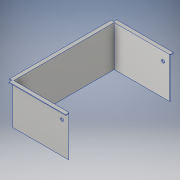
# Autodesk Inventor part: Intake Drop
Saved by Autodesk Inventor 2017 (Build 210142000, 142)
## iProperties
Created: 2020-02-19
Part Number: Intake Drop
Material: Aluminum 6061
Document SubType Name: Modeling
Designer: S346553810
Density: 2.7 g/cm^3
Appearance: Aluminum - Flat
Author: S346553810
Autodesk Inventor part; units mm, degrees
ref_plane "YZ Plane" through (0, 0, 0) normal (1, 0, 0) x (0, 1, 0)
ref_plane "XZ Plane" through (0, 0, 0) normal (0, 1, 0) x (-1, 0, 0)
ref_plane "XY Plane" through (0, 0, 0) normal (0, 0, 1) x (1, 0, 0)
sketch "Sketch1" plane through (0, 0, 0) normal (0, 1, 0) x (-1, 0, 0)
  line L0 (-115.8875, -209.55) -> (115.8875, -209.55)
  line L1 (115.8875, -209.55) -> (115.8875, 209.55)
  line L2 (115.8875, 209.55) -> (-115.8875, 209.55)
  line L3 (-115.8875, -209.55) -> (115.8875, 209.55) construction
  line L4 (115.8875, -209.55) -> (-115.8875, 209.55) construction
  line L5 (113.3475, 207.01) -> (113.3475, -207.01)
  line L6 (113.3475, -207.01) -> (-113.3475, -207.01)
  line L7 (-113.3475, 207.01) -> (113.3475, 207.01)
  line L8 (-113.3475, 207.01) -> (-115.8875, 209.55)
  line L9 (-113.3475, -207.01) -> (-115.8875, -209.55)
  point P0 (0, 0)
  dimension "d0" = 231.775
  dimension "d1" = 419.1
  dimension "d2" = 2.54
  constraints: 20 end point, 3 perpendicular, 2 midpoint, 2 parallel, 1 horizontal, 1 other
  measures "d0" distance of L2.end L1.end
  measures "d1" distance of L1.end L0.end
  measures "d2" distance between parallel lines of L1 L5
extrude "Extrusion1" add sketch "Sketch1" along normal blind 127
sketch "Sketch2" plane through (0, 127, 0) normal (0, 1, 0) x (1, 0, 0)
  line L0 (-115.8875, -209.55) -> (-128.5875, -209.55)
  line L1 (-128.5875, -209.55) -> (-128.5875, 209.55)
  line L2 (-128.5875, 209.55) -> (-115.8875, 209.55)
  line L3 (-115.8875, 209.55) -> (-115.8875, -209.55)
  line L4 (-115.8875, 209.55) -> (115.8875, 209.55)
  line L5 (115.8875, 209.55) -> (115.8875, 222.25)
  line L6 (115.8875, 222.25) -> (-115.8875, 222.25)
  line L7 (-115.8875, 222.25) -> (-115.8875, 209.55)
  line L8 (-115.8875, -209.55) -> (115.8875, -209.55) projected
  line L9 (115.8875, -209.55) -> (-115.8875, -209.55)
  line L10 (-115.8875, -209.55) -> (-115.8875, -222.25)
  line L11 (-115.8875, -222.25) -> (115.8875, -222.25)
  line L12 (115.8875, -222.25) -> (115.8875, -209.55)
  point P0 (0, 0)
  dimension "d5" = 12.7
  dimension "d6" = 419.1
  dimension "d7" = 231.775
  dimension "d8" = 12.7
  dimension "d9" = 12.7
  dimension "d12" = 231.775
  constraints: 24 end point, 6 parallel, 3 horizontal, 3 perpendicular, 1 point on line
  measures "d5" distance of L1.end L2.end
  measures "d6" distance of L0.end L1.end
  measures "d7" distance of L6.end L5.end
  measures "d8" distance of L5.end L4.end
  measures "d9" distance of L10.end L9.end
  measures "d12" distance of L10.end L11.end
extrude "Extrusion2" add sketch "Sketch2" against normal blind 2.54
sketch "Sketch3" plane through (0, 0, 0) normal (0, -1, 0) x (1, 0, 0)
  line L0 (115.8875, -209.55) -> (-115.8875, -209.55) projected
  line L1 (113.3475, -207.01) -> (115.8875, -209.55) projected
  line L2 (-113.3475, -207.01) -> (113.3475, -207.01) projected
  line L3 (-113.3475, 207.01) -> (-113.3475, -207.01) projected
  line L4 (113.3475, 207.01) -> (-113.3475, 207.01) projected
  line L5 (115.8875, 209.55) -> (113.3475, 207.01) projected
  line L6 (-115.8875, 209.55) -> (115.8875, 209.55) projected
  line L7 (-115.8875, -209.55) -> (-115.8875, 209.55) projected
  point P0 (0, 0)
extrude "Extrusion3" add sketch "Sketch3" along normal blind 40.64
sketch "Sketch4" plane through (115.8875, 124.46, -209.55) normal (0, 0, -1) x (-1, 0, 0)
  circle A0 centre (27.94, -34.925) radius 6.35
  line L0 (0, 0) -> (0, -165.1) projected
  line L1 (231.775, 0) -> (0, 0) projected
  circle A1 centre (85.3615, -107.95) radius 99.06 construction
  point P0 (115.8875, -124.46)
  dimension "d15" = 12.7
  dimension "d25" = 27.94
  dimension "d26" = 34.925
  constraints: 1 centre point
  measures "d15" diameter of A0
  measures "d25" distance from line of L0 A0.centre
  measures "d26" distance from line of A0.centre L1
extrude "Extrusion4" cut sketch "Sketch4" against normal through all
sketch "Sketch5" plane through (-115.8875, 127, -209.55) normal (0, 0, -1) x (-1, 0, 0)
  line L0 (5.08, -2.54) -> (5.08, 49.46) projected
  line L1 (0, 0) -> (0, -2.54) projected
  line L2 (2.54, -2.54) -> (2.54, -27.94) projected
  line L3 (0, -2.54) -> (0, 0) projected
  line L4 (0, 0) -> (2.54, 0)
  line L5 (2.54, 0) -> (2.54, -2.54)
  line L6 (2.54, -2.54) -> (0, -2.54)
  line L7 (0, -2.54) -> (0, 0)
  point P0 (-115.8875, -127)
  constraints: 8 end point, 2 parallel, 1 horizontal, 1 perpendicular
extrude "Extrusion5" add sketch "Sketch5" along normal blind 12.7
sketch "Sketch6" plane through (0, 127, 0) normal (0, 1, 0) x (1, 0, 0)
  line L0 (-115.8875, -209.55) -> (-128.5875, -209.55) projected
  line L1 (-115.8875, -209.55) -> (-118.4275, -209.55)
  line L2 (-118.4275, -209.55) -> (-118.4275, -222.25)
  line L3 (-118.4275, -222.25) -> (-115.8875, -222.25)
  line L4 (-115.8875, -222.25) -> (-115.8875, -209.55)
  point P0 (0, 0)
  dimension "d20" = 2.54
  constraints: 8 end point, 2 parallel, 1 horizontal, 1 perpendicular
  measures "d20" distance of L3.end L2.end
extrude "Extrusion6" add sketch "Sketch6" against normal blind 2.54
body "Solid1"
